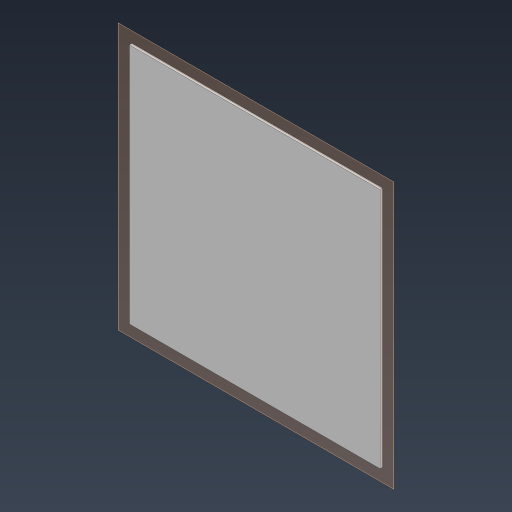
# Autodesk Inventor part: Задняя панель
Saved by Autodesk Inventor 2023.2 (Build 272271030, 271C)
## iProperties
Created: 2025-08-26
Part Number: Задняя панель
Material: Типовые
Document SubType Name: Modeling
Designer: Олег Коноваленко
Density: 1 g/cm^3
Appearance: По умолчанию
Author: Олег Коноваленко
Autodesk Inventor part; units mm, degrees
ref_plane "YZ Plane" through (0, 0, 0) normal (1, 0, 0) x (0, 1, 0)
ref_plane "XZ Plane" through (0, 0, 0) normal (0, 1, 0) x (-1, 0, 0)
sketch "Эскиз1" plane through (0, 0, 0) normal (0, 0, 1) x (1, 0, 0)
  line L0 (200, -193) -> (-200, -193)
  line L1 (-200, -193) -> (-200, 193)
  line L2 (-200, 193) -> (200, 193)
  line L3 (200, 193) -> (200, -193)
  line L4 (200, -193) -> (-200, 193) construction
  line L5 (-200, -193) -> (200, 193) construction
  point P0 (0, 0)
  dimension "d0" = 400
  dimension "d1" = 386
  constraints: 12 end point, 2 midpoint, 2 parallel, 1 horizontal, 1 perpendicular
  measures "d0" distance of L0.start L0.end
  measures "d1" distance of L0.end L1.end
extrude "Выдавливание1" add sketch "Эскиз1" along normal mid plane 4
